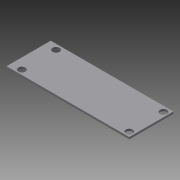
# Autodesk Inventor part: PCB
Saved by Autodesk Inventor 2015 (Build 190159000, 159)
## iProperties
Created: 2017-02-11
Part Number: PCB
Material: Generic
Document SubType Name: Modeling
Designer: stran
Density: 1 g/cm^3
Appearance: Default
Author: stran
Autodesk Inventor part; units mm, degrees
ref_plane "YZ Plane" through (0, 0, 0) normal (1, 0, 0) x (0, 1, 0)
ref_plane "XZ Plane" through (0, 0, 0) normal (0, 1, 0) x (-1, 0, 0)
ref_plane "XY Plane" through (0, 0, 0) normal (0, 0, 1) x (1, 0, 0)
sketch "Sketch1" plane through (0, 0, 0) normal (0, 1, 0) x (-1, 0, 0)
  line L0 (0, 0) -> (66.03, 0)
  line L1 (66.03, 0) -> (66.03, -23.8)
  line L2 (66.03, -23.8) -> (0, -23.8)
  line L3 (0, -23.8) -> (0, 0)
  dimension "d0" = 66.03
  dimension "d1" = 23.8
  constraints: 8 end point, 2 parallel, 1 horizontal, 1 perpendicular
  measures "d0" distance of L0.start L0.end
  measures "d1" distance of L2.end L0.start
extrude "Extrusion1" add sketch "Sketch1" along normal blind 1.0583
sketch "Sketch2" plane through (0, 1.0583, 0) normal (0, 1, 0) x (1, 0, 0)
  line L0 (0, 0) -> (0, 23.8) projected
  line L1 (-66.03, 0) -> (0, 0) projected
  point P0 (-60.325, 2.54)
  point P1 (-2.54, 2.54)
  point P2 (-2.54, 20.955)
  point P3 (-60.325, 20.955)
  dimension "d4" = 60.325
  dimension "d5" = 60.325
  dimension "d6" = 2.54
  dimension "d7" = 2.54
  dimension "d8" = 2.54
  dimension "d9" = 2.54
  dimension "d10" = 20.955
  dimension "d11" = 20.955
  measures "d4" distance from line of L0 point (-60.325, 2.54)
  measures "d5" distance from line of L0 point (-60.325, 20.955)
  measures "d6" distance from line of L1 point (-60.325, 2.54)
  measures "d7" distance from line of L1 point (-2.54, 2.54)
  measures "d8" distance from line of L0 point (-2.54, 2.54)
  measures "d9" distance from line of L0 point (-2.54, 20.955)
  measures "d10" distance from line of L1 point (-2.54, 20.955)
  measures "d11" distance from line of L1 point (-60.325, 20.955)
hole "Hole1" at (-60.325, 1.0583, -2.54) at (-2.54, 1.0583, -2.54) at (-2.54, 1.0583, -20.955) at (-60.325, 1.0583, -20.955) direction (0, -1, 0) diameter 3.81 end through all
equation "\"d5\" = d4"
equation "\"d7\" = d6"
equation "\"d8\" = d7"
equation "\"d9\" = d8"
equation "\"d11\" = d10"
body "Solid1"
